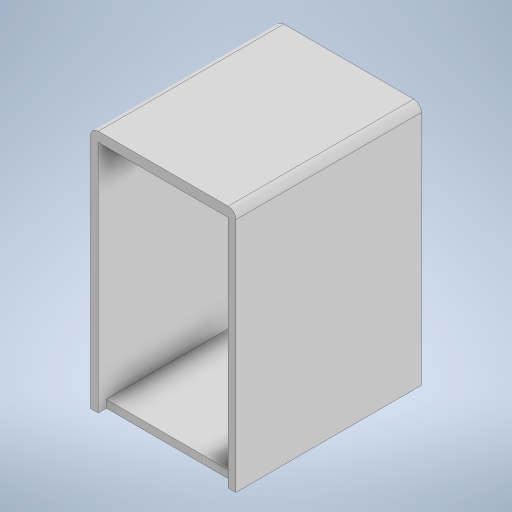
# Autodesk Inventor part: Base_Demo_1
Saved by Autodesk Inventor 2023.5 (Build 275446020, 446B)
## iProperties
Created: 2025-04-11
Part Number: Base_Demo_1
Material: Generic
Document SubType Name: Modeling
Designer: Lucky
Density: 1 g/cm^3
Appearance: Default
Author: Lucky
Autodesk Inventor part; units mm, degrees
ref_plane "YZ Plane" through (0, 0, 0) normal (1, 0, 0) x (0, 1, 0)
ref_plane "XZ Plane" through (0, 0, 0) normal (0, 1, 0) x (-1, 0, 0)
ref_plane "XY Plane" through (0, 0, 0) normal (0, 0, 1) x (1, 0, 0)
sketch "Sketch3" plane through (0, 0, 0) normal (0, 0, 1) x (1, 0, 0)
  line L0 (0, 0) -> (33.6, 0)
  line L1 (33.6, 0) -> (33.6, 58.6)
  line L2 (33.6, 58.6) -> (0, 58.6)
  line L3 (0, 58.6) -> (0, 0)
  line L4 (-2, 60.6) -> (35.6, 60.6)
  line L5 (35.6, 60.6) -> (35.6, -2)
  line L6 (35.6, -2) -> (-2, -2)
  line L7 (-2, -2) -> (-2, 60.6)
  dimension "d36" = 33.6
  dimension "d37" = 58.6
  dimension "d38" = 2
  constraints: 16 end point, 4 parallel, 2 perpendicular, 1 horizontal, 3 other
  measures "d36" distance of L2.end L1.end
  measures "d37" distance between parallel lines of L0 L2
  measures "d38" distance between parallel lines of L2 L4
extrude "Extrusion3" add sketch "Sketch3" along normal blind 46
sketch "Sketch4" plane through (0, 0, 0) normal (0, 0, -1) x (-1, 0, 0)
  circle A0 centre (-16.775, 44.825) radius 13.5
  line L0 (0, 58.6) -> (-33.6, 58.6) projected
  line L1 (0, 0) -> (0, 58.6) projected
  line L2 (-33.6, 58.6) -> (-33.6, 0) projected
  line L3 (-33.6, 6.5) -> (0, 6.5)
  line L4 (0, 0) -> (0, 58.6) projected
  line L5 (-33.6, 0) -> (0, 0) projected
  line L6 (-33.6, 0) -> (0, 0) projected
  line L7 (-33.6, 6.5) -> (0, 6.5)
  line L8 (0, 6.5) -> (0, 0)
  line L9 (0, 0) -> (-33.6, 0)
  line L10 (-33.6, 0) -> (-33.6, 6.5)
  line L11 (-35.6, 60.6) -> (2, 60.6) projected
  line L12 (2, 60.6) -> (2, -2) projected
  line L13 (-35.6, 60.6) -> (2, 60.6)
  line L14 (2, 60.6) -> (2, -2)
  line L15 (2, -2) -> (-35.6, -2)
  line L16 (-35.6, -2) -> (-35.6, 60.6)
  line L17 (-33.6, 58.6) -> (-33.6, 0) projected
  line L18 (-33.6, 0) -> (-33.6, -2)
  line L19 (0, 0) -> (0, -2)
  line L20 (2, -2) -> (-35.6, -2) projected
  point P0 (0, 6.5)
  dimension "d41" = 27
  dimension "d42" = 13.775
  dimension "d43" = 16.775
  dimension "d44" = 6.5
  constraints: 22 end point, 5 parallel, 5 point on line, 3 perpendicular, 2 horizontal, 1 centre point
  measures "d41" diameter of A0
  measures "d42" distance from line of L0 A0.centre
  measures "d43" distance from line of L1 A0.centre
  measures "d44" distance between parallel lines of L5 L3
extrude "Extrusion4" add sketch "Sketch4" along normal blind 2 contours L1 L3 L2 L0 | L0 L2 L18 L15 L16 L11 L12 L19 L1
sketch "Sketch5" plane through (-2, 60.6, 46) normal (0, 1, 0) x (1, 0, 0)
  line L0 (0, 0) -> (37.6, 0) projected
  line L1 (37.6, 48) -> (37.6, 0) projected
  line L2 (0, 0) -> (37.6, 0)
  line L3 (37.6, 0) -> (37.6, 48)
  line L4 (37.6, 48) -> (0, 48)
  line L5 (0, 48) -> (0, 0)
  point P0 (2, 46)
  constraints: 8 end point, 2 parallel, 1 horizontal, 1 perpendicular
extrude "Extrusion5" add sketch "Sketch5" along normal blind 0.5
sketch "Sketch6" plane through (0, 0, 46) normal (0, 0, 1) x (1, 0, 0)
  line L0 (-2, -2) -> (35.6, -2)
  line L1 (35.6, -2) -> (35.6, 6.3)
  line L2 (35.6, 6.3) -> (-2, 6.3)
  line L3 (-2, 6.3) -> (-2, -2)
  line L4 (0, 6.5) -> (0, -2) projected
  line L5 (0, 6.3) -> (0, -2)
  line L6 (35.6, -2) -> (33.6, -2) projected
  line L7 (33.6, 6.3) -> (33.6, -2)
  point P0 (0, 0)
  dimension "d56" = 8.3
  constraints: 12 end point, 4 point on line, 3 perpendicular, 2 parallel, 1 horizontal
  measures "d56" distance between parallel lines of L0 L2
extrude "Extrusion6" cut sketch "Sketch6" against normal blind 2.1 contours L4 L2 L7 L0
sketch "Sketch7" plane through (-2, -2, -2) normal (-1, 0, 0) x (0, 0, 1)
  line L0 (0, 37.3) -> (6, 37.3)
  line L1 (0, 24.3) -> (6, 24.3)
  line L2 (6, 37.3) -> (6, 24.3)
  line L3 (2, 33.325) -> (2, 60.325) projected
  line L4 (48, 0) -> (0, 0) projected
  line L5 (2, 37.3) -> (2, 24.3)
  line L6 (0, 37.3) -> (0, 24.3)
  line L7 (0, 33.325) -> (0, 60.325) projected
  point P0 (2, 2)
  point P1 (3, 24.3)
  point P2 (2, 37.3)
  dimension "d59" = 6
  dimension "d60" = 13
  dimension "d61" = 24.3
  constraints: 10 end point, 2 horizontal, 2 point on line, 1 collinear, 1 midpoint, 1 parallel, 1 perpendicular
  measures "d59" distance of L0.end L0.start
  measures "d60" distance from line of point (3, 24.3) L0
  measures "d61" distance between parallel lines of L4 L1
extrude "Extrusion7" cut sketch "Sketch7" against normal up to surface (2 mm away) contours L0 L2 L1 L5 L3
fillet "Fillet3" radius 2 1 edges at (35.6, 61.1, 22)
fillet "Fillet4" radius 2 1 edges at (-2, 61.1, 22)
body "Solid2"
